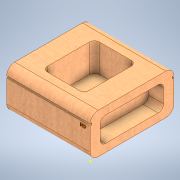
# Autodesk Inventor part: PassengerSectionGBR
Saved by Autodesk Inventor 2020.1 (Build 241239000, 239)
## iProperties
Created: 2020-02-27
Part Number: PassengerSectionGBR
Material: Generic
Document SubType Name: Modeling
Designer: super
Density: 1 g/cm^3
Appearance: Cherry - Natural Low Gloss
Author: super
Autodesk Inventor part; units mm, degrees
ref_plane "YZ Plane" through (0, 0, 0) normal (1, 0, 0) x (0, 1, 0)
ref_plane "XZ Plane" through (0, 0, 0) normal (0, 1, 0) x (-1, 0, 0)
ref_plane "XY Plane" through (0, 0, 0) normal (0, 0, 1) x (1, 0, 0)
sketch "Sketch1" plane through (0, 0, 0) normal (0, 1, 0) x (-1, 0, 0)
  point P0 (0, 0)
sketch "Sketch2" plane through (0, 0, 0) normal (0, 1, 0) x (-1, 0, 0)
  line L0 (0, 0) -> (80.518, 0)
  line L1 (80.518, 0) -> (80.518, -80.518)
  line L2 (80.518, -80.518) -> (0, -80.518)
  line L3 (0, -80.518) -> (0, 0)
  dimension "d0" = 80.518
  dimension "d1" = 80.518
  constraints: 8 end point, 2 parallel, 1 horizontal, 1 perpendicular
  measures "d0" distance of L1.end L2.end
  measures "d1" distance of L0.end L1.end
extrude "Extrusion1" add sketch "Sketch2" along normal blind 38.862
fillet "Fillet1" radius 7.62 4 edges at (-40.259, 0, 0) (-40.259, 38.862, 0) (-40.259, 0, -80.518) (-40.259, 38.862, -80.518)
sketch "Sketch3" plane through (0, 38.862, 0) normal (0, 1, 0) x (1, 0, 0)
  line L0 (-80.518, 80.518) -> (0, 80.518) projected
  line L1 (0, 7.62) -> (0, 72.898) projected
  line L2 (-20.828, 65.278) -> (-61.214, 65.278)
  line L3 (-61.214, 65.278) -> (-61.214, 14.986)
  line L4 (-61.214, 14.986) -> (-20.828, 14.986)
  line L5 (-20.828, 14.986) -> (-20.828, 65.278)
  point P0 (0, 0)
  dimension "d7" = 40.386
  dimension "d8" = 50.292
  constraints: 8 end point, 2 parallel, 1 horizontal, 1 perpendicular
  measures "d7" distance of L4.end L3.end
  measures "d8" distance of L3.end L2.end
extrude "Extrusion2" cut sketch "Sketch3" against normal blind 27.178
fillet "Fillet2" radius 5.08 4 edges at (-61.214, 25.273, -14.986) (-61.214, 25.273, -65.278) (-20.828, 25.273, -14.986) (-20.828, 25.273, -65.278)
sketch "Sketch4" plane through (0, 0, -7.62) normal (1, 0, 0) x (0, 0, -1)
  line L0 (72.898, 7.62) -> (72.898, 31.242) projected
  line L1 (62.992, 31.242) -> (2.032, 31.242)
  line L2 (2.032, 31.242) -> (2.032, 7.62)
  line L3 (2.032, 7.62) -> (62.992, 7.62)
  line L4 (62.992, 7.62) -> (62.992, 31.242)
  point P0 (-7.62, 0)
  dimension "d12" = 9.906
  dimension "d13" = 60.96
  dimension "d14" = 23.622
  constraints: 8 end point, 2 parallel, 1 horizontal, 1 perpendicular
  measures "d12" distance of L0.end L1.start
  measures "d13" distance of L3.end L2.end
  measures "d14" distance of L2.end L1.end
extrude "Extrusion3" cut sketch "Sketch4" against normal blind 14.478
fillet "Fillet3" radius 5.08 4 edges at (-7.239, 31.242, -9.652) (-7.239, 7.62, -9.652) (-7.239, 7.62, -70.612) (-7.239, 31.242, -70.612)
sketch "Sketch5" plane through (0, 31.242, -80.518) normal (0, 0, -1) x (-1, 0, 0)
  line L0 (0, 0) -> (0, -5.08) projected
  line L1 (0, 0) -> (0, -1.524)
  line L2 (0, -1.524) -> (80.518, -1.524)
  line L3 (80.518, -23.622) -> (80.518, 0) projected
  line L4 (80.518, 0) -> (0, 0) projected
  line L5 (80.518, 0) -> (0, 0)
  point P0 (0, -31.242)
  dimension "d18" = 1.524
  constraints: 6 end point, 2 point on line, 1 collinear, 1 perpendicular
  measures "d18" distance of L0.start L1.end
extrude "Extrusion4" cut sketch "Sketch5" against normal blind 1.524
sketch "Sketch6" plane through (-80.518, 31.242, 0) normal (0, 0, 1) x (1, 0, 0)
  line L0 (0, 0) -> (0, 7.62) projected
  line L1 (0, 0) -> (0, -1.524)
  line L2 (0, -23.622) -> (0, 0) projected
  line L3 (0, -1.524) -> (80.518, -1.524) projected
  line L4 (0, -1.524) -> (80.518, -1.524)
  line L5 (80.518, -5.08) -> (80.518, 0) projected
  line L6 (80.518, -1.524) -> (80.518, 0)
  line L7 (80.518, 0) -> (0, 0) projected
  line L8 (80.518, 0) -> (0, 0)
  point P0 (80.518, -31.242)
  dimension "d21" = 1.524
  constraints: 8 end point, 2 collinear, 1 perpendicular, 1 point on line
  measures "d21" distance of L0.start L1.end
extrude "Extrusion5" cut sketch "Sketch6" against normal blind 1.524
sketch "Sketch7" plane through (-80.518, 0, -72.898) normal (-1, 0, 0) x (0, 0, 1)
  arc A0 (72.898, 31.242) -> (65.278, 38.862) centre (65.278, 31.242) ccw projected
  line L0 (64.2238, 32.0041) -> (0.7238, 32.0041)
  line L1 (0.7238, 32.0041) -> (0.7238, 6.6041)
  line L2 (0.7238, 6.6041) -> (64.2238, 6.6041)
  line L3 (64.2238, 6.6041) -> (64.2238, 32.0041)
  point P0 (72.898, 0)
  dimension "d26" = 63.5
  dimension "d27" = 25.4
  constraints: 8 end point, 2 parallel, 1 horizontal, 1 perpendicular
  measures "d26" distance of L2.end L1.end
  measures "d27" distance of L1.end L0.end
extrude "Extrusion6" cut sketch "Sketch7" against normal blind 14.478
fillet "Fillet4" radius 5.08 4 edges at (-73.279, 32.0041, -72.1742) (-73.279, 6.6041, -72.1742) (-73.279, 6.6041, -8.6742) (-73.279, 32.0041, -8.6742)
sketch "Sketch8" plane through (-80.518, 7.62, 0) normal (0, 0, 1) x (1, 0, 0)
  line L0 (71.0966, 20.5879) -> (80.9129, 20.5879) construction
  line L1 (80.9129, 20.5879) -> (80.9129, 15.2848) construction
  line L2 (80.9129, 15.2848) -> (71.0966, 15.2848) construction
  line L3 (71.0966, 15.2848) -> (71.0966, 20.5879) construction
  line L4 (74.0186, 17.4781) -> (73.6135, 17.4781)
  line L5 (73.6135, 17.4781) -> (73.6135, 20.1038)
  line L6 (73.6135, 20.1038) -> (72.8182, 18.3179)
  line L7 (72.8182, 18.3179) -> (72.5712, 18.3179)
  line L8 (72.5712, 18.3179) -> (71.7832, 20.1038)
  line L9 (71.7832, 20.1038) -> (71.7832, 17.4781)
  line L10 (71.7832, 17.4781) -> (71.4053, 17.4781)
  line L11 (71.4053, 17.4781) -> (71.4053, 20.5261)
  line L12 (71.4053, 20.5261) -> (71.9586, 20.5261)
  line L13 (71.9586, 20.5261) -> (72.7194, 18.8292)
  line L14 (72.7194, 18.8292) -> (73.4554, 20.5261)
  line L15 (73.4554, 20.5261) -> (74.0186, 20.5261)
  line L16 (74.0186, 20.5261) -> (74.0186, 17.4781)
  spline S0 degree 2 poles (74.4657, 19.5357) (74.4657, 19.7703) (74.6188, 20.1606) (74.7522, 20.3014) knots 0 0 0 1 2 2 2
  spline S1 degree 2 poles (74.7522, 20.3014) (74.8782, 20.4372) (75.2462, 20.5879) (75.4339, 20.5879) knots 0 0 0 1 2 2 2
  spline S2 degree 2 poles (75.4339, 20.5879) (75.6439, 20.5879) (75.9847, 20.4471) (76.1107, 20.3137) knots 0 0 0 1 2 2 2
  spline S3 degree 2 poles (76.1107, 20.3137) (76.2688, 20.1457) (76.4417, 19.6023) (76.4417, 19.1849) knots 0 0 0 1 2 2 2
  spline S4 degree 2 poles (76.4417, 19.1849) (76.4417, 18.807) (76.2713, 18.1302) (76.1058, 17.9054) knots 0 0 0 1 2 2 2
  spline S5 degree 2 poles (76.1058, 17.9054) (75.9304, 17.6683) (75.4364, 17.4189) (75.0758, 17.4189) knots 0 0 0 1 2 2 2
  spline S6 degree 2 poles (75.0758, 17.4189) (74.9943, 17.4189) (74.809, 17.4361) (74.73, 17.4608) knots 0 0 0 1 2 2 2
  line L17 (74.73, 17.4608) -> (74.73, 17.8536)
  line L18 (74.73, 17.8536) -> (74.7497, 17.8536)
  spline S7 degree 2 poles (74.7497, 17.8536) (74.8016, 17.8239) (75.019, 17.7721) (75.1301, 17.7721) knots 0 0 0 1 2 2 2
  spline S8 degree 2 poles (75.1301, 17.7721) (75.5302, 17.7721) (75.9872, 18.3006) (76.0193, 18.7897) knots 0 0 0 1 2 2 2
  spline S9 degree 2 poles (76.0193, 18.7897) (75.8563, 18.6786) (75.5599, 18.5773) (75.3845, 18.5773) knots 0 0 0 1 2 2 2
  spline S10 degree 2 poles (75.3845, 18.5773) (75.2166, 18.5773) (74.9374, 18.6514) (74.7967, 18.7576) knots 0 0 0 1 2 2 2
  spline S11 degree 2 poles (74.7967, 18.7576) (74.6336, 18.8836) (74.4657, 19.2664) (74.4657, 19.5357) knots 0 0 0 1 2 2 2
  spline S12 degree 2 poles (76.0292, 19.2763) (76.0292, 19.5851) (75.9156, 19.9753) (75.8143, 20.0815) knots 0 0 0 1 2 2 2
  spline S13 degree 2 poles (75.8143, 20.0815) (75.7254, 20.1803) (75.5401, 20.2544) (75.4314, 20.2544) knots 0 0 0 1 2 2 2
  spline S14 degree 2 poles (75.4314, 20.2544) (75.1795, 20.2544) (74.8806, 19.8938) (74.8806, 19.5529) knots 0 0 0 1 2 2 2
  spline S15 degree 2 poles (74.8806, 19.5529) (74.8806, 19.3603) (74.9794, 19.1108) (75.0881, 19.0219) knots 0 0 0 1 2 2 2
  spline S16 degree 2 poles (75.0881, 19.0219) (75.1672, 18.9577) (75.3623, 18.9157) (75.4759, 18.9157) knots 0 0 0 1 2 2 2
  spline S17 degree 2 poles (75.4759, 18.9157) (75.6068, 18.9157) (75.9082, 19.0071) (76.0218, 19.0836) knots 0 0 0 1 2 2 2
  spline S18 degree 2 poles (76.0218, 19.0836) (76.0243, 19.1133) (76.0292, 19.2146) (76.0292, 19.2763) knots 0 0 0 1 2 2 2
  point P0 (80.518, -7.62)
  constraints: 2 other
sketch "Sketch9" plane through (-80.518, 7.62, 0) normal (0, 0, 1) x (1, 0, 0)
  point P0 (80.518, -7.62)
emboss "Emboss1" sketch "Sketch8" operation add depth 0.508 direction (0, 0, -1)
body "Solid1"
